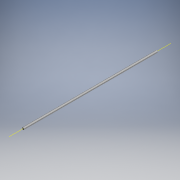
# Autodesk Inventor part: 12 Inch Hex Axle
Saved by Autodesk Inventor 2019 (Build 230136000, 136)
## iProperties
Part Number: 12 Inch Hex Axle
Material: Generic
Document SubType Name: Modeling
Designer: Delta
Appearance: Default
Author: Delta
Autodesk Inventor part; units mm, degrees
ref_plane "YZ Plane" through (0, 0, 0) normal (1, 0, 0) x (0, 1, 0)
ref_plane "XZ Plane" through (0, 0, 0) normal (0, 1, 0) x (-1, 0, 0)
ref_plane "XY Plane" through (0, 0, 0) normal (0, 0, 1) x (1, 0, 0)
sketch "Sketch1" plane through (0, 0, 0) normal (0, 0, 1) x (1, 0, 0)
  circle A0 centre (0, 0) radius 2.8829
  line L0 (-0.2691, 2.8703) -> (2.4206, 1.3174)
  line L1 (-0.2691, 2.8703) -> (2.8368, 2.8703) construction
  line L2 (2.4206, 1.3174) -> (2.4206, -1.5658)
  line L3 (2.4206, -1.5658) -> (0, -2.8829)
  line L4 (0, -2.8829) -> (-2.4966, -1.4416)
  line L5 (-2.4966, -1.4416) -> (-2.4966, 1.4416)
  line L6 (-0.2691, 2.8703) -> (-2.4966, 1.4416)
  dimension "d0" = 5.7658
  dimension "d1" = 30
  dimension "d2" = 120
  dimension "d3" = 2.8831
  dimension "d7" = 2.8831
  constraints: 14 end point, 5 point on circle, 1 centre point, 1 coincident, 1 equal length, 1 horizontal, 1 vertical
  measures "d0" diameter of A0
  measures "d1" angle of L0 L1
  measures "d2" angle of L0 L2
  measures "d3" distance of L0.end L2.end
  measures "d7" distance of L4.end L5.end
extrude "Extrusion1" add sketch "Sketch1" along normal blind 355.6 contours L0 L2 L3 L4 L5 L6
fillet "Fillet1" radius 0.1 12 edges at (1.0758, 2.0939, 355.6) (-1.3828, 2.1559, 355.6) (-2.4966, 0, 355.6) (-1.2483, -2.1622, 355.6) (1.2103, -2.2243, 355.6) (2.4206, -0.1242, 355.6) (1.0758, 2.0939, 0) (-1.3828, 2.1559, 0) (-2.4966, 0, 0) (-1.2483, -2.1622, 0) (1.2103, -2.2243, 0) (2.4206, -0.1242, 0)
equation "\"d7\" = d3"
body "Solid1"
